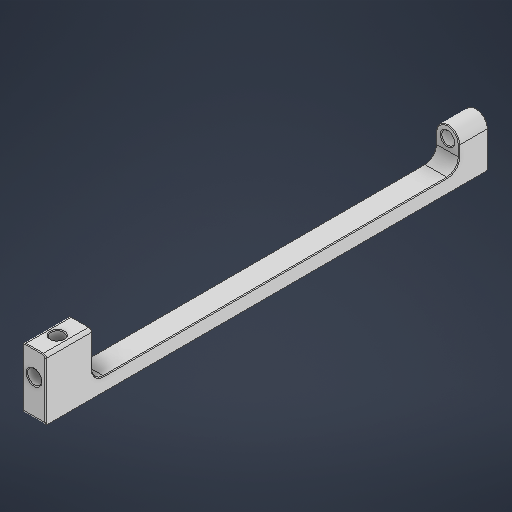
# Autodesk Inventor part: Half-Shaft-Motor
Saved by Autodesk Inventor 2025 (Build 290162010, 162A)
## iProperties
Created: 2025-12-05
Part Number: Half-Shaft-Motor
Material: Generic
Document SubType Name: Modeling
Designer: FizzyApple12
Density: 1 g/cm^3
Appearance: Default
Author: FizzyApple12
Autodesk Inventor part; units mm, degrees
ref_plane "YZ Plane" through (0, 0, 0) normal (1, 0, 0) x (0, 1, 0)
ref_plane "XZ Plane" through (0, 0, 0) normal (0, 1, 0) x (-1, 0, 0)
ref_plane "XY Plane" through (0, 0, 0) normal (0, 0, 1) x (1, 0, 0)
sketch "Sketch1" plane through (0, 0, 0) normal (0, 0, 1) x (1, 0, 0)
  circle A0 centre (0, 0) radius 2.5
  line L0 (-4, -7.6487) -> (4, -7.6487)
  line L1 (4, -7.6487) -> (4, -12.6487)
  line L2 (4, -12.6487) -> (-4, -12.6487)
  line L3 (-4, -12.6487) -> (-4, -7.6487)
  line L4 (0, 0) -> (0, -7.6487) construction
  line L5 (-4, -7.6487) -> (4, -7.6487)
  line L6 (4, -7.6487) -> (4, 4)
  line L7 (4, 4) -> (-4, 4)
  line L8 (-4, 4) -> (-4, -7.6487)
  line L9 (0, 0) -> (0, 4) construction
  line L10 (-4, 4) -> (4, 4)
  line L11 (4, 4) -> (4, 8.5)
  line L12 (4, 8.5) -> (-4, 8.5)
  line L13 (-4, 8.5) -> (-4, 4)
  circle A1 centre (0, 0) radius 2.25
  point P0 (0, 2.5)
  dimension "d0" = 5
  dimension "d1" = 8
  dimension "d2" = 5
  dimension "d3" = 4
  dimension "d18" = 6
  dimension "d30" = 4.5
  constraints: 28 end point, 6 parallel, 3 coincident, 3 horizontal, 3 perpendicular, 2 midpoint, 1 centre point, 1 point on line, 1 vertical, 1 vertical alignment, 2 other
  measures "d1" distance of L1.end L2.end
  measures "d2" distance of L0.end L1.end
  measures "d3" distance of L4.start L9.end
  measures "d18" distance from line of L12 point (0, 2.5)
  measures "d30" diameter of A1
extrude "Extrusion1" add sketch "Sketch1" against normal blind 16 contours L8 L7 L6 L0 | L0 L1 L2 L3 | L13 L12 L11 L7
extrude "Extrusion2" add sketch "Sketch1" against normal blind 152.3335 contours L0 L1 L2 L3
extrude "Extrusion3" add sketch "Sketch1" along normal blind 10 from surface at -152.3335 contours A0 | L8 L7 L6 L0 | L0 L1 L2 L3 | A1
sketch "Sketch2" plane through (0, 0, -152.3335) normal (0, 0, -1) x (-1, 0, 0)
  point P0 (0, 0)
  point P1 (0, 0)
hole "Hole1" at (0, 0, -152.3335) direction (0, 0, 1) diameter 4.5 depth 12 tip angle 118
sketch "Sketch3" plane through (-4, 8.5, 0) normal (0, 1, 0) x (1, 0, 0)
  line L0 (8, 0) -> (0, 0) construction
  line L1 (8, 0) -> (8, 16) construction
  line L2 (0, 16) -> (8, 16) construction
  line L3 (0, 0) -> (0, 16) construction
  line L4 (0, 0) -> (0, 16) construction
  line L5 (8, 16) -> (0, 0) construction
  point P0 (4, 0)
  point P1 (4, 8)
  constraints: 2 end point, 1 midpoint
hole "Hole2" at (0, 8.5, -8) direction (0, -1, 0) diameter 3.4 depth 9 tip angle 118 counterbore diameter 4.5 counterbore depth 5 clearance for "Socket Head Cap Screw" size "M3" standard "Ansi Metric M Profile"
extrude "Extrusion4" add sketch "Sketch1" against normal blind 0.5 from surface at -152.3335 contours A0
fillet "Fillet1" radius 4 4 edges at (4, 4, -147.3335) (-4, 4, -147.3335) (0, -7.6487, -16) (0, -7.6487, -142.3335)
fillet "Fillet2" radius 1 4 edges at (4, 8.5, -8) (-4, 8.5, -8) (0, -12.6487, 0) (0, -12.6487, -152.3335)
chamfer "Chamfer1" distance 0.25 angle 45 39 edges at (4, -5.8243, -152.3335) (-2.8285, 2.8285, -152.3335) (0, 4, -152.3335) (2.8285, 2.8285, -152.3335) (-4, -5.8243, -152.3335) (-4, -12.3558, -152.0406) (-4, -12.6487, -76.1667) (-4, -12.3558, -0.2929) (-4, -2.0744, 0) (-3.7071, 8.2071, 0) (0, 8.5, 0) (3.7071, 8.2071, 0) (4, -2.0744, 0) (4, -12.3558, -0.2929) (4, -12.6487, -76.1667) (4, -12.3558, -152.0406) (0, -2.25, -142.3335) (-2.8285, 2.8285, -142.3335) (0, 4, -142.3335) (2.8285, 2.8285, -142.3335) (4, -1.8244, -142.3335) (4, -6.4772, -141.162) (4, -7.6487, -79.1667) (4, -6.4772, -17.1715) (4, 1.9256, -16) (3.7071, 8.2071, -16) (0, 8.5, -16) (-3.7071, 8.2071, -16) (-4, 1.9256, -16) (-4, -6.4772, -17.1715) (-4, -7.6487, -79.1667) (-4, -6.4772, -141.162) (-4, -1.8244, -142.3335) (-2.5, 0, -16) (-2.5, 0, 0) (0, 8.5, -10.25) (-0.0091, 2.5, -9.7) (0, 3.5, -9.7) (-2.5, 0, -152.3335)
body "Solid1"
